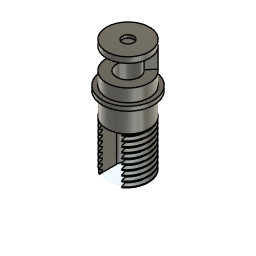
SingleAxisTestJig v4 (Autodesk Fusion 360 archive; units mm, degrees)
design "Initial axle design"
Autodesk Fusion 360 part; units mm, degrees
sketch "Sketch15" plane through (0, 0, 0) normal (0, 0, 1) x (1, 0, 0)
  circle A0 centre (0, 0) radius 15
  dimension "d33" = 30
  constraint coincident A0.centre origin
  measures "d33" diameter of A0
extrude "Extrude10" add sketch "Sketch15" along normal blind 33
thread "Thread2" "ISO Metric profile 30.0 M30x3.5 6g" major diameter 29.7345 minor diameter 25.732 pitch 3.5 angle 60 modelled right hand crest width 0.4992 on face at (14.9255, -1.4935, 22) crest through (14.8673, 0, -0.875)
sketch "Sketch24" plane through (0, 0, 0) normal (0, 0, -1) x (1, 0, 0)
  spline S0 degree 3 poles (-7.4686, 10.4764) (-8.918, 9.5987) (-10.1792, 8.4429) (-12.2244, 5.6786) (-12.9736, 4.0859) (-13.8402, 0.6575) (-13.9314, -1.1495) (-13.418, -4.7469) (-12.8001, -6.4997) (-11.2234, -9.1838) (-10.4366, -10.1892) (-8.6068, -11.9859) (-7.5677, -12.7651) (-6.4407, -13.3997) knots 0 0 0 0 0.508319 0.508319 1.030956 1.030956 1.567907 1.567907 2.119164 2.119164 2.499584 2.499584 2.886551 2.886551 2.886551 2.886551
  arc A0 (-6.4407, -13.3997) -> (6.4407, -13.3997) centre (0, 0) ccw
  spline S1 degree 3 poles (6.4407, -13.3997) (8.1035, -12.4634) (9.5698, -11.2151) (11.9044, -8.2591) (12.7645, -6.5914) (13.775, -3.0641) (13.9333, -1.2438) (13.5396, 2.306) (13.0097, 4.0031) (11.6093, 6.567) (10.9224, 7.5086) (9.3334, 9.1701) (8.4424, 9.8867) (7.4686, 10.4764) knots 0 0 0 0 0.572495 0.572495 1.130652 1.130652 1.674465 1.674465 2.203926 2.203926 2.552907 2.552907 2.895334 2.895334 2.895334 2.895334
  arc A1 (7.4686, 10.4764) -> (-7.4686, 10.4764) centre (0, 0) ccw
move_body "Move1" bodies 1 to x (-1, 0, 0) y (0, -1, 0) z (0, 0, 1) at (0, 0, 0)
sketch "Sketch16" plane through (0, 0, 0) normal (0, 0, -1) x (1, 0, 0)
  spline S0 degree 3 poles (7.4686, -10.4764) (8.918, -9.5987) (10.1792, -8.4429) (12.2244, -5.6786) (12.9736, -4.0859) (13.8402, -0.6575) (13.9314, 1.1495) (13.418, 4.7469) (12.8001, 6.4997) (11.2234, 9.1838) (10.4366, 10.1892) (8.6068, 11.9859) (7.5677, 12.7651) (6.4407, 13.3997) knots 0 0 0 0 0.508319 0.508319 1.030956 1.030956 1.567907 1.567907 2.119164 2.119164 2.499584 2.499584 2.886551 2.886551 2.886551 2.886551
  arc A0 (6.4407, 13.3997) -> (-6.4407, 13.3997) centre (0, 0) ccw
  spline S1 degree 3 poles (-6.4407, 13.3997) (-8.1035, 12.4634) (-9.5698, 11.2151) (-11.9044, 8.2591) (-12.7645, 6.5914) (-13.775, 3.0641) (-13.9333, 1.2438) (-13.5396, -2.306) (-13.0097, -4.0031) (-11.6093, -6.567) (-10.9224, -7.5086) (-9.3334, -9.1701) (-8.4424, -9.8867) (-7.4686, -10.4764) knots 0 0 0 0 0.572495 0.572495 1.130652 1.130652 1.674465 1.674465 2.203926 2.203926 2.552907 2.552907 2.895334 2.895334 2.895334 2.895334
  arc A1 (-7.4686, -10.4764) -> (7.4686, -10.4764) centre (0, 0) ccw
  circle A2 centre (0, 0) radius 8
  line L0 (-8, 0) -> (8, 0)
  line L1 (8, 0) -> (8, 15)
  line L2 (8, 15) -> (-8, 15)
  line L3 (-8, 15) -> (-8, 0)
  dimension "d38" = 16
  dimension "d39" = 16
  dimension "d40" = 15
  constraint coincident A0.centre A1.centre
  constraint horizontal L0
  constraint vertical L1
  constraint horizontal L2
  constraint vertical L3
  constraint coincident A2 L0.start
  measures "d38" diameter of A2
  measures "d39" distance of L0.start L0.end
  measures "d40" distance of L0.start L2.end
extrude "Extrude11" cut sketch "Sketch16" against normal blind 33 contours S0 A0 S1 A2 L1 L3 | S0 A0 S1 L1 L2 L3 | A2 L0 | A2 L0
sketch "Sketch17" plane through (0, 0, 33) normal (0, 0, 1) x (-1, 0, 0)
  line L0 (-8, 0) -> (-8, 10.6536)
  spline S0 degree 3 poles (-0.0111, -14.8672) (1.8933, -14.7451) (3.756, -14.2566) (7.142, -12.6063) (8.6405, -11.4769) (11.0814, -8.7374) (12.0138, -7.1661) (13.1993, -3.797) (13.4582, -2.0381) (13.3089, 0.8796) (13.0986, 2.026) (12.3878, 4.2124) (11.896, 5.2446) (11.2745, 6.1984) knots 0 0 0 0 0.572495 0.572495 1.130652 1.130652 1.674465 1.674465 2.203926 2.203926 2.552907 2.552907 2.895334 2.895334 2.895334 2.895334
  arc A0 (11.2745, 6.1984) -> (8, 10.0764) centre (0, 0) ccw
  spline S1 degree 3 poles (-8, 10.6536) (-9.1394, 9.9204) (-10.1623, 9.0157) (-12.1843, 6.5975) (-13.0505, 5.009) (-14.1488, 1.5451) (-14.3526, -0.3023) (-14.0966, -3.4047) (-13.824, -4.6519) (-12.9549, -7.0645) (-12.3568, -8.2175) (-11.6168, -9.2782) knots 0.623383 0.623383 0.623383 0.623383 1.030956 1.030956 1.567907 1.567907 2.119164 2.119164 2.499584 2.499584 2.886551 2.886551 2.886551 2.886551
  arc A1 (-11.6168, -9.2782) -> (-0.0111, -14.8672) centre (0, 0) ccw
  line L1 (8, 10.0764) -> (8, 0)
  arc A2 (-8, 0) -> (8, 0) centre (0, 0) ccw
  circle A3 centre (0, 0) radius 15
  dimension "d43" = 30
  constraint concentric A0 A3
  measures "d43" diameter of A3
extrude "Extrude12" add sketch "Sketch17" along normal blind 16 contours L0 S0 A0 S1 A1 L1 A2 | A3
sketch "Sketch18" plane through (0, 0, 49) normal (0, 0, 1) x (-1, 0, 0)
  circle A0 centre (0, 0) radius 15
  circle A1 centre (0, 0) radius 18
  dimension "d46" = 36
  constraint coincident A0.centre A1.centre
  measures "d46" diameter of A1
extrude "Extrude13" add sketch "Sketch18" along normal blind 3 contours A0 | A1
sketch "Sketch19" plane through (0, 0, 52) normal (0, 0, 1) x (-1, 0, 0)
  circle A0 centre (0, 0) radius 18
  circle A1 centre (0, 0) radius 15
  dimension "d49" = 30
  constraint concentric A0 A1
  measures "d49" diameter of A1
extrude "Extrude14" add sketch "Sketch19" along normal blind 9 contours A1
sketch "Sketch20" plane through (0, 0, 33) normal (0, 0, -1) x (1, 0, 0)
  circle A0 centre (0, 0) radius 15
  arc A1 (-8, 10.0764) -> (-11.2745, 6.1984) centre (0, 0) ccw
  spline S0 degree 3 poles (8, 10.6536) (9.1394, 9.9204) (10.1623, 9.0157) (12.1843, 6.5975) (13.0505, 5.009) (14.1488, 1.5451) (14.3526, -0.3023) (14.0966, -3.4047) (13.824, -4.6519) (12.9549, -7.0645) (12.3568, -8.2175) (11.6168, -9.2782) knots 0.623383 0.623383 0.623383 0.623383 1.030956 1.030956 1.567907 1.567907 2.119164 2.119164 2.499584 2.499584 2.886551 2.886551 2.886551 2.886551
  arc A2 (0.0111, -14.8672) -> (11.6168, -9.2782) centre (0, 0) ccw
  line L0 (-8, 10.0764) -> (-8, 0)
  arc A3 (-8, 0) -> (8, 0) centre (0, 0) ccw
  line L1 (8, 0) -> (8, 10.6536)
  spline S1 degree 3 poles (0.0111, -14.8672) (-1.8933, -14.7451) (-3.756, -14.2566) (-7.142, -12.6063) (-8.6405, -11.4769) (-11.0814, -8.7374) (-12.0138, -7.1661) (-13.1993, -3.797) (-13.4582, -2.0381) (-13.3089, 0.8796) (-13.0986, 2.026) (-12.3878, 4.2124) (-11.896, 5.2446) (-11.2745, 6.1984) knots 0 0 0 0 0.572495 0.572495 1.130652 1.130652 1.674465 1.674465 2.203926 2.203926 2.552907 2.552907 2.895334 2.895334 2.895334 2.895334
  circle A4 centre (0, 0) radius 8
  dimension "d52" = 16
  constraint concentric A0 A4
  measures "d52" diameter of A4
extrude "Extrude15" cut sketch "Sketch20" against normal blind 28 contours A3 A4
sketch "Sketch21" plane through (0, 0, 0) normal (1, 0, 0) x (0, 1, 0)
  line L0 (15, 61) -> (8, 61)
  line L1 (8, 61) -> (8, 76)
  line L2 (8, 76) -> (15, 76)
  line L3 (15, 76) -> (15, 61)
  constraint horizontal L0
  constraint vertical L1
  constraint horizontal L2
  constraint vertical L3
revolve "Revolve2" add sketch "Sketch21" angle 40 about axis through (0, 0, 1.75) along (0, 0, -1) second angle 40
sketch "Sketch22" plane through (0, 0, 76) normal (0, 0, 1) x (-1, 0, 0)
  arc A0 (-5.1423, -6.1284) -> (5.1423, -6.1284) centre (0, 0) ccw
  line L0 (-5.1423, -6.1284) -> (-9.6418, -11.4907)
  arc A1 (-9.6418, -11.4907) -> (9.6418, -11.4907) centre (0, 0) ccw
  line L1 (9.6418, -11.4907) -> (5.1423, -6.1284)
  circle A2 centre (0, 0) radius 15
  dimension "d57" = 30
  constraint concentric A0 A2
  measures "d57" diameter of A2
extrude "Extrude16" add sketch "Sketch22" along normal blind 4
sketch "Sketch23" plane through (0, 0, 80) normal (0, 0, 1) x (-1, 0, 0)
  circle A0 centre (0, 0) radius 15
  circle A1 centre (0, 0) radius 4
  dimension "d60" = 8
  constraint concentric A0 A1
  measures "d60" diameter of A1
extrude "Extrude17" cut sketch "Sketch23" against normal blind 2 contours A1

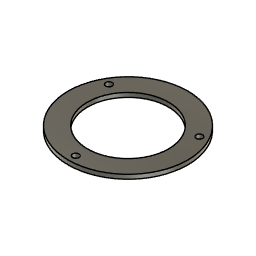
design "Top bearing retainer"
Autodesk Fusion 360 part; units mm, degrees
sketch "Sketch1" plane through (0, 0, 0) normal (0, 0, 1) x (1, 0, 0)
  circle A0 centre (0, 0) radius 28
  circle A1 centre (0, 0) radius 19
  dimension "d1" = 56
  dimension "d2" = 38
  constraint coincident A0.centre A1.centre
  constraint concentric A0 A1
  measures "d1" diameter of A0
  measures "d2" diameter of A1
extrude "Extrude1" add sketch "Sketch1" along normal blind 2
sketch "Sketch2" plane through (0, 0, 2) normal (0, 0, 1) x (-1, 0, 0)
  circle A0 centre (0, 0) radius 19
  circle A1 centre (0, 0) radius 28
  circle A2 centre (0, 24.5) radius 1.5
  dimension "d5" = 3
  measures "d5" diameter of A2
extrude "Extrude2" cut sketch "Sketch2" against normal blind 2 contours A2
pattern_circular "C-Pattern1" count 3 over 360 about axis through (0, 0, 1.75) along (0, 0, 1) of 1 faces at (-1.4925, -24.3506, 0.6667)
